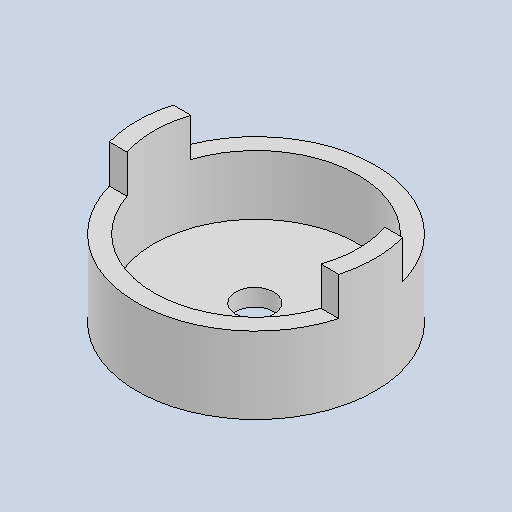
# Autodesk Inventor part: magneticslotV1
Saved by Autodesk Inventor 2022 (Build 260153000, 153)
## iProperties
Created: 2021-06-03
Part Number: magneticslotV1
Material: Generic
Document SubType Name: Modeling
Designer: User
Density: 1 g/cm^3
Appearance: Default
Author: User
Autodesk Inventor part; units mm, degrees
ref_plane "YZ Plane" through (0, 0, 0) normal (1, 0, 0) x (0, 1, 0)
ref_plane "XZ Plane" through (0, 0, 0) normal (0, 1, 0) x (-1, 0, 0)
ref_plane "XY Plane" through (0, 0, 0) normal (0, 0, 1) x (1, 0, 0)
sketch "Sketch1" plane through (0, 0, 0) normal (0, 1, 0) x (-1, 0, 0)
  circle A0 centre (0, 0) radius 14
  circle A1 centre (0, 0) radius 12
  dimension "d0" = 28
  dimension "d1" = 24
  constraints: 2 centre point, 2 coincident
  measures "d0" diameter of A0
  measures "d1" diameter of A1
extrude "Extrusion1" add sketch "Sketch1" along normal blind 7
sketch "Sketch2" plane through (0, 7, 0) normal (0, 1, 0) x (1, 0, 0)
  line L0 (14, -3.75) -> (-14, -3.75)
  line L1 (-14, -3.75) -> (-14, 3.75)
  line L2 (-14, 3.75) -> (14, 3.75)
  line L3 (14, 3.75) -> (14, -3.75)
  line L4 (14, -3.75) -> (-14, 3.75) construction
  line L5 (-14, -3.75) -> (14, 3.75) construction
  line L6 (-0.5, 5) -> (0.5, 5)
  line L7 (0.5, 5) -> (0.5, -5)
  line L8 (0.5, -5) -> (-0.5, -5)
  line L9 (-0.5, -5) -> (-0.5, 5)
  line L10 (-0.5, 5) -> (0.5, -5) construction
  line L11 (0.5, 5) -> (-0.5, -5) construction
  circle A0 centre (0, 0) radius 12
  circle A1 centre (0, 0) radius 14
  point P0 (0, 0)
  point P1 (-13.4884, 3.75)
  point P2 (-13.4884, -3.75)
  point P3 (-11.399, -3.75)
  point P4 (-11.399, 3.75)
  point P5 (13.4884, 3.75)
  point P6 (11.399, 3.75)
  point P7 (11.399, -3.75)
  point P8 (13.4884, -3.75)
  dimension "d4" = 28
  dimension "d5" = 7.5
  dimension "d27" = 24
  dimension "d28" = 28
  constraints: 24 end point, 4 midpoint, 4 parallel, 2 centre point, 2 coincident, 2 horizontal, 2 perpendicular
  measures "d4" distance of L1.end L2.end
  measures "d5" distance of L0.end L1.end
  measures "d27" diameter of A0
  measures "d28" diameter of A1
sketch "Sketch3" plane through (0, 0, 0) normal (0, -1, 0) x (1, 0, 0)
  circle A0 centre (0, 0) radius 14
  dimension "d17" = 28
  constraints: 1 centre point, 1 coincident
  measures "d17" diameter of A0
extrude "Extrusion3" add sketch "Sketch3" along normal blind 2
sketch "Sketch5" plane through (0, 0, 0) normal (0, 1, 0) x (1, 0, 0)
  point P0 (0, 0)
  point P1 (-0.0372, -0.1116)
hole "Hole2" at (-0.0372, 0, 0.1116) direction (0, -1, 0) diameter 4.5 end through all clearance for "Hex Head Machine Screw" size "M4" standard "Ansi Metric M Profile"
extrude "Extrusion4" add sketch "Sketch2" along normal blind 4.5 contours L0 A0 L2 A1 | A1 L2 A0 L0
body "Solid1"
